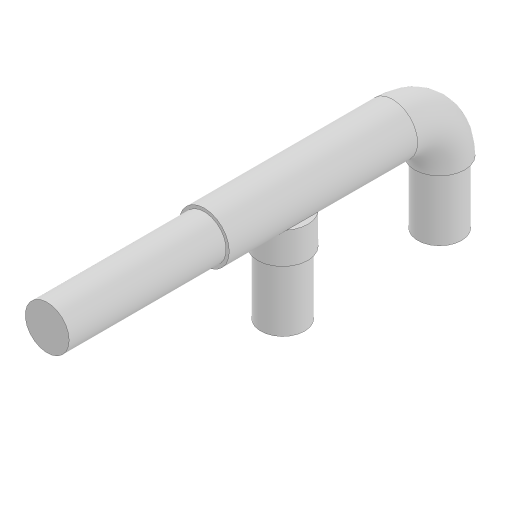
# Autodesk Inventor part: 1p10 DP3 roller attachment final
Saved by Autodesk Inventor 2023 (Build 270158000, 158)
## iProperties
Created: 2023-02-17
Part Number: 1p10 DP3 roller attachment final
Material: Generic
Document SubType Name: Modeling
Designer: Ethan Ko
Density: 1 g/cm^3
Appearance: Default
Author: Ethan Ko
Autodesk Inventor part; units mm, degrees
ref_plane "YZ Plane" through (0, 0, 0) normal (1, 0, 0) x (0, 1, 0)
sketch "Sketch2" plane through (0, 0, 0) normal (0, 0, 1) x (1, 0, 0)
  circle A0 centre (0, 0) radius 4
  dimension "d0" = 8
  constraints: 1 centre point, 1 coincident
  measures "d0" diameter of A0
ref_plane "Work Plane1" through (0, -7.5, 0) normal (0, 1, 0) x (-1, 0, 0)
sketch "Sketch3" plane through (0, -7.5, 0) normal (0, 1, 0) x (-1, 0, 0)
  circle A0 centre (0, -7.5) radius 4
  line L0 (5.6, 0) -> (-5.6, 0) projected
  point P0 (0, 0)
  dimension "d2" = 8
  dimension "d3" = 7.5
  constraints: 1 centre point
  measures "d2" diameter of A0
  measures "d3" distance of point (0, 0) A0.centre
revolve "Revolution1" add sketch "Sketch3" angle 90 about axis through (-10, -7.5, 0) along (1, 0, 0)
extrude "Extrusion1" add sketch "Sketch2" along normal blind 17.5
sketch "Sketch4" plane through (0, 0, 17.5) normal (0, 0, 1) x (1, 0, 0)
  circle A0 centre (0, 0) radius 4
  dimension "d7" = 8
  constraints: 1 centre point, 1 coincident
  measures "d7" diameter of A0
ref_plane "Work Plane2" through (0, 0, 17.5) normal (0, 0, 1) x (1, 0, 0)
extrude "Extrusion2" add sketch "Sketch4" along normal blind 12.5
sketch "Sketch5" plane through (0, -7.5, 0) normal (0, 1, 0) x (-1, 0, 0)
  circle A0 centre (0, 17.5) radius 4
  line L0 (-10.5, 17.5) -> (10.5, 17.5) projected
  point P0 (0, 0)
  dimension "d11" = 8
  dimension "d12" = 0
  constraints: 1 centre point
  measures "d11" diameter of A0
  measures "d12" distance from line of L0 A0.centre
extrude "Extrusion3" add sketch "Sketch5" along normal blind 5
sketch "Sketch7" plane through (0, -7.5, -7.5) normal (0, -1, 0) x (1, 0, 0)
  circle A0 centre (0, 0) radius 3.5
  point P0 (0, 7.5)
  dimension "d18" = 7
  constraints: 1 centre point
  measures "d18" diameter of A0
extrude "Extrusion4" add sketch "Sketch7" along normal blind 10
sketch "Sketch8" plane through (0, -7.5, 0) normal (0, -1, 0) x (1, 0, 0)
  circle A0 centre (0, 17.5) radius 3.5
  circle A1 centre (0, -7.5) radius 3.5 projected
  point P0 (0, 0)
  dimension "d21" = 7
  dimension "d22" = 25
  constraints: 1 centre point
  measures "d21" diameter of A0
  measures "d22" distance of A1.centre A0.centre
extrude "Extrusion5" add sketch "Sketch8" along normal blind 10 contours A0
sketch "Sketch10" plane through (0, 0, 30) normal (0, 0, 1) x (1, 0, 0)
  circle A0 centre (0, 0) radius 4 projected
  circle A1 centre (0, 0) radius 3.5
  dimension "d29" = 7
  constraints: 1 centre point, 1 coincident
  measures "d29" diameter of A1
extrude "Extrusion7" add sketch "Sketch10" along normal mid plane 50 contours A1
body "Solid1"
